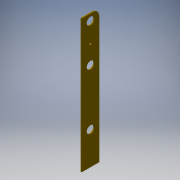
# Autodesk Inventor part: Back Plate
Saved by Autodesk Inventor 2017 (Build 210142000, 142)
## iProperties
Created: 2017-01-13
Part Number: Back Plate
Material: Generic
Document SubType Name: Modeling
Designer: Ben
Density: 1 g/cm^3
Appearance: Gold
Author: Ben
Autodesk Inventor part; units mm, degrees
ref_plane "YZ Plane" through (0, 0, 0) normal (1, 0, 0) x (0, 1, 0)
ref_plane "XZ Plane" through (0, 0, 0) normal (0, 1, 0) x (-1, 0, 0)
ref_plane "XY Plane" through (0, 0, 0) normal (0, 0, 1) x (1, 0, 0)
sketch "Sketch1" plane through (0, 0, 0) normal (1, 0, 0) x (0, 1, 0)
  line L0 (386.842, -25.4) -> (0, -25.4) construction
  circle A0 centre (94.742, -25.4) radius 11.1125
  circle A1 centre (367.792, -25.4) radius 11.1125
  circle A2 centre (256.667, -25.4) radius 11.1125
  circle A3 centre (310.642, -25.4) radius 3.175
  line L1 (0, 0) -> (386.842, 0)
  line L2 (386.842, 0) -> (386.842, -50.8)
  line L3 (386.842, -50.8) -> (0, -50.8)
  line L4 (0, -50.8) -> (0, 0)
  line L5 (76.2, -9.525) -> (107.95, -9.525) construction
  line L6 (107.95, -9.525) -> (107.95, -41.275) construction
  circle A4 centre (107.95, -9.525) radius 1.27
  circle A5 centre (107.95, -41.275) radius 1.27
  circle A6 centre (76.2, -9.525) radius 1.27
  dimension "d3" = 22.225
  dimension "d4" = 273.05
  dimension "d9" = 161.925
  dimension "d12" = 6.35
  dimension "d13" = 57.15
  dimension "d15" = 50.8
  dimension "d16" = 19.05
  dimension "d17" = 94.742
  dimension "d18" = 2.54
  dimension "d19" = 9.525
  dimension "d20" = 31.75
  dimension "d21" = 76.2
  constraints: 14 end point, 7 centre point, 4 equal radius, 4 point on line, 3 coincident, 3 perpendicular, 2 horizontal, 2 midpoint, 2 parallel
  measures "d3" diameter of A0
  measures "d4" distance of A0.centre A1.centre
  measures "d9" distance of A0.centre A2.centre
  measures "d12" diameter of A3
  measures "d13" distance of A1.centre A3.centre
  measures "d15" distance of L3.end L1.start
  measures "d16" distance from line of L2 A1.centre
  measures "d17" distance from line of L4 A0.centre
  measures "d18" diameter of A4
  measures "d19" distance between parallel lines of L1 L5
  measures "d20" distance of L5.start L5.end
  measures "d21" distance from line of L4 L5.start
extrude "Extrusion1" add sketch "Sketch1" along normal blind 3.175
fillet "Fillet1" radius 19.05 1 edges at (1.5875, 386.842, -50.8)
body "Solid1"
